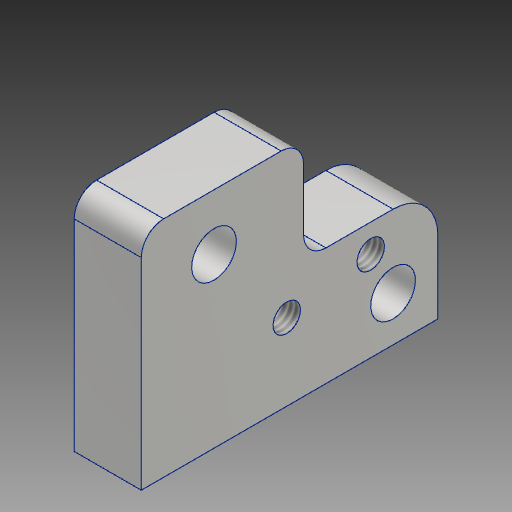
# Autodesk Inventor part: Dribbler Lagerbock
Saved by Autodesk Inventor 2019.4 (Build 234330000, 330)
## iProperties
Part Number: Dribbler Lagerbock
Material: Aluminium 6061
Document SubType Name: Modeling
Designer: rYan
Mass: 5.82991 g
Surface Area: 16.945 cm^2
Volume: 2.15922 cm^3
Density: 2.7 g/cm^3
Appearance: Aluminium - flach
Author: rYan
Autodesk Inventor part; units mm, degrees
ref_plane "YZ Plane" through (0, 0, 0) normal (1, 0, 0) x (0, 1, 0)
ref_plane "XZ Plane" through (0, 0, 0) normal (0, 1, 0) x (-1, 0, 0)
ref_plane "XY Plane" through (0, 0, 0) normal (0, 0, 1) x (1, 0, 0)
sketch "Skizze1" plane through (0, 0, 0) normal (1, 0, 0) x (0, 1, 0)
  line L0 (5.5, 0) -> (32, 0)
  line L1 (32, 0) -> (32, 10.5)
  line L2 (5.5, 20) -> (5.5, 0)
  line L3 (5.5, 20) -> (20, 20)
  line L4 (20, 20) -> (20, 10.5)
  line L5 (32, 10.5) -> (20, 10.5)
  circle A0 centre (12, 15) radius 0.5
  circle A1 centre (28, 4) radius 0.5
  circle A2 centre (26, 8) radius 0.5
  line L6 (0, 24) -> (0, -4) projected
  line L7 (-6.4, 0) -> (38.4, 0) projected
  dimension "d1" = 10.5
  dimension "d3" = 20
  dimension "d21" = 1
  dimension "d28" = 1
  dimension "d31" = 4
  dimension "d41" = 1
  dimension "d43" = 8
  dimension "d54" = 5.5
  dimension "d55" = 26
  dimension "d56" = 28
  dimension "d61" = 15
  dimension "d62" = 12
  dimension "d127" = 32
  dimension "d128" = 14.5
  constraints: 12 end point, 3 centre point, 2 parallel, 1 collinear, 1 horizontal, 1 perpendicular, 1 vertical
  measures "d1" distance of L0.end L1.end
  measures "d3" distance between parallel lines of L0 L3
  measures "d21" diameter of A0
  measures "d28" diameter of A1
  measures "d31" distance from line of A1.centre L0
  measures "d41" diameter of A2
  measures "d43" distance from line of L0 A2.centre
  measures "d54" distance between parallel lines of L6 L2
  measures "d55" distance from line of L6 A2.centre
  measures "d56" distance from line of L6 A1.centre
  measures "d61" distance from line of L0 A0.centre
  measures "d62" distance from line of L6 A0.centre
  measures "d127" distance between parallel lines of L1 L6
  measures "d128" distance of L2.start L3.end
extrude "Extrusion1" add sketch "Skizze1" along normal mid plane 6
sketch "Skizze9" plane through (-3, 0, 0) normal (-1, 0, 0) x (0, 0, 1)
  circle A0 centre (8, 26) radius 0.5 projected
  point P0 (0, 0)
  constraints: 1 coincident
hole "Feder" at (-3, 26, 8) direction (1, 0, 0) diameter 2.459 end through all thread size "M3x0.5" class "6H" standard "ISO Metric profile"
sketch "Skizze3" plane through (-3, 0, 0) normal (-1, 0, 0) x (0, 0, 1)
  circle A0 centre (4, 28) radius 0.5 projected
  constraints: 1 coincident
hole "Dribbler" at (-3, 28, 4) direction (1, 0, 0) diameter 4 end through all
sketch "Skizze4" plane through (-3, 0, 0) normal (-1, 0, 0) x (0, 0, 1)
  circle A0 centre (15, 12) radius 0.5 projected
  circle A1 centre (15, 12) radius 0.5 projected
  point P0 (0, 0)
  constraints: 1 coincident
hole "Chipper" at (-3, 12, 15) direction (1, 0, 0) diameter 4 end through all
sketch "Skizze5" plane through (3, 32, 0) normal (0, 0, -1) x (-1, 0, 0)
  line L0 (0, 0) -> (6, 0) projected
  line L1 (0, -26.5) -> (0, 0) projected
  line L2 (6, -26.5) -> (0, -26.5) projected
  line L3 (6, 0) -> (6, -26.5) projected
  line L4 (3, -26.5) -> (3, 0) construction
  point P0 (3, -10)
  point P1 (3, -24)
  point P2 (3, -17)
  point P3 (3, -13.25)
  dimension "d58" = 7
  dimension "d89" = 7
  dimension "d97" = 2.5
  constraints: 3 midpoint, 3 point on line, 2 end point
  measures "d58" distance of point (3, -17) point (3, -10)
  measures "d89" distance of point (3, -17) point (3, -24)
  measures "d97" distance from line of L2 point (3, -24)
hole "Montage" at (0, 22, 0) at (0, 8, 0) at (0, 15, 0) direction (0, 0, 1) diameter 2.459 depth 7 tip angle 118 thread size "M3x0.5" class "6H" standard "ISO Metric profile"
fillet "Rundung2" radius 2 3 edges at (0, 5.5, 20) (0, 20, 20) (0, 20, 10.5)
fillet "Rundung3" radius 4 1 edges at (0, 32, 10.5)
sketch "Skizze6" plane through (-3, 0, 0) normal (-1, 0, 0) x (0, 0, 1)
  line L0 (0, 13.7705) -> (0, 16.2295) projected
  line L1 (7, 16.2295) -> (7, 13.7705) projected
  line L2 (0, 20.7705) -> (0, 23.2295) projected
  line L3 (7, 23.2295) -> (7, 20.7705) projected
  circle A0 centre (15, 12) radius 2 projected
  line L4 (7, 13.7705) -> (7, 23.2295) construction
  line L5 (7, 13.7705) -> (0, 13.7705) construction
  line L6 (0, 23.2295) -> (0, 13.7705) construction
  line L7 (0, 5.5) -> (0, 32) construction
  line L8 (7, 18.5) -> (0, 18.5) construction
  line L9 (15, 12) -> (15, 7) construction
  line L10 (0, 6.7705) -> (0, 9.2295) projected
  line L11 (7, 9.2295) -> (7, 6.7705) projected
  line L12 (7, 6.7705) -> (7, 16.2295) construction
  line L13 (7, 6.7705) -> (0, 6.7705) construction
  line L14 (0, 6.7705) -> (0, 16.2295) construction
  line L15 (7, 11.5) -> (0, 11.5) construction
  point P0 (0, 0)
  point P1 (3.5, 11.5)
  point P2 (3.5, 18.5)
  point P3 (7.7388, 8)
  point P4 (3.5, 11.5)
  dimension "d71" = 5
  constraints: 14 end point, 6 midpoint, 2 perpendicular, 2 vertical, 1 coincident, 1 parallel, 1 other
  measures "d71" distance of L9.start L9.end
hole "Bohrung4" [suppressed]
sketch "Skizze8" plane through (-3, 0, 0) normal (-1, 0, 0) x (0, 0, 1)
  line L0 (21, 16) -> (21, 9) construction
  line L1 (-4.2, 0) -> (25.2, 0) projected
  line L2 (0, 38.4) -> (0, -6.4) projected
  point P0 (0, 0)
  dimension "d72" = 7
  dimension "d73" = 9
  dimension "d74" = 21
  constraints: 2 coincident, 2 end point, 1 vertical
  measures "d72" distance of L0.start L0.end
  measures "d73" distance from line of L1 point (21, 9)
  measures "d74" distance between parallel lines of L2 L0
hole "Bohrung5" [suppressed]
sketch "Skizze10" plane through (-3, 0, 0) normal (-1, 0, 0) x (0, 0, 1)
  line L0 (0, 13.7705) -> (0, 16.2295) projected
  line L1 (7, 16.2295) -> (7, 13.7705) projected
  line L2 (0, 6.7705) -> (0, 9.2295) projected
  line L3 (7, 9.2295) -> (7, 6.7705) projected
  line L4 (-4, 0) -> (24, 0) projected
  line L5 (0, 38.4) -> (0, -6.4) projected
  point P0 (0, 0)
  point P1 (6.85, 18.5)
  dimension "d98" = 18.5
  dimension "d99" = 6.85
  measures "d98" distance from line of L4 point (6.85, 18.5)
  measures "d99" distance from line of L5 point (6.85, 18.5)
hole "Alternativer Anschlag" at (-3, 18.5, 6.85) direction (1, 0, 0) diameter 2.459 end through all thread size "M3x0.5" class "6H" standard "ISO Metric profile"
